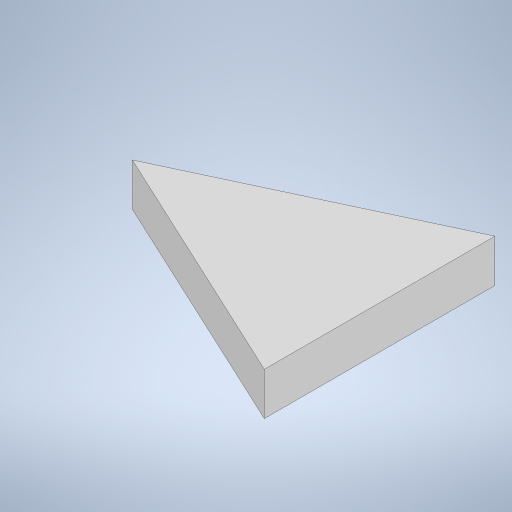
# Autodesk Inventor part: Tri_Box
Saved by Autodesk Inventor 2024.3 (Build 283343000, 343)
## iProperties
Created: 2025-06-26
Part Number: Tri_Box
Material: Generic
Document SubType Name: Modeling
Designer: 1
Density: 1 g/cm^3
Appearance: Default
Author: 1
Autodesk Inventor part; units mm, degrees
ref_plane "YZ Plane" through (0, 0, 0) normal (1, 0, 0) x (0, 1, 0)
ref_plane "XZ Plane" through (0, 0, 0) normal (0, 1, 0) x (-1, 0, 0)
ref_plane "XY Plane" through (0, 0, 0) normal (0, 0, 1) x (1, 0, 0)
sketch "Sketch1" plane through (0, 0, 0) normal (0, 1, 0) x (-1, 0, 0)
  line L0 (75.2034, 0) -> (-34.7966, 51.2938)
  line L1 (-34.7966, 51.2938) -> (-34.7966, -51.2938)
  line L2 (-34.7966, -51.2938) -> (75.2034, 0)
  line L3 (97.2034, 0) -> (-56.7966, 0) projected
  line L4 (63.3724, 0) -> (-29.7966, 43.4454)
  line L5 (-29.7966, 43.4454) -> (-29.7966, -43.4454)
  line L6 (-29.7966, -43.4454) -> (63.3724, 0)
  point P0 (0, 0)
  dimension "d0" = 50
  dimension "d1" = 110
  dimension "d2" = 5
  dimension "d3" = 5
  constraints: 12 end point, 2 parallel, 2 vertical, 1 point on line, 1 other
  measures "d0" angle of L2 L0
  measures "d1" distance from line of L0.start L1
  measures "d2" distance between parallel lines of L0 L4
  measures "d3" distance between parallel lines of L1 L5
extrude "Extrusion1" add sketch "Sketch1" along normal blind 17 contours L3 L4 L5 L1 L0 | L2 L1 L3 L5 L6
sketch "Sketch2" plane through (0, 17, 0) normal (0, 1, 0) x (1, 0, 0)
  line L0 (34.7966, 51.2938) -> (-75.2034, 0) projected
  line L1 (-75.2034, 0) -> (34.7966, -51.2938) projected
  line L2 (34.7966, -51.2938) -> (34.7966, 51.2938) projected
  point P0 (0, 0)
extrude "Extrusion2" add sketch "Sketch2" along normal blind 2
body "Solid1"
